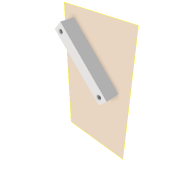
# Autodesk Inventor part: NematostellaImager_mirrormount
Saved by Autodesk Inventor 2022.5 (Build 265521000, 521)
## iProperties
Created: 2023-11-06
Part Number: NematostellaImager_mirrormount
Material: Generisch
Document SubType Name: Modeling
Designer: diederichbenedict
Density: 1 g/cm^3
Appearance: Vorgabe
Author: diederichbenedict
Autodesk Inventor part; units mm, degrees
ref_plane "YZ Plane" through (0, 0, 0) normal (1, 0, 0) x (0, 1, 0)
ref_plane "XZ Plane" through (0, 0, 0) normal (0, 1, 0) x (-1, 0, 0)
ref_plane "XY Plane" through (0, 0, 0) normal (0, 0, 1) x (1, 0, 0)
ref_plane "Arbeitsebene1" through (0, 0, 0) normal (0, 0, 1) x (1, 0, 0)
sketch "Skizze1" plane through (0, 0, 0) normal (0, 0, 1) x (1, 0, 0)
  line L0 (-0.2844, 28.5315) -> (-56.8529, 85.1) projected
  circle A0 centre (-11.3693, 45.2732) radius 1.49 projected
  circle A1 centre (-41.3693, 75.2732) radius 1.4 projected
  line L1 (-47.0261, 75.2732) -> (-41.3693, 80.9301)
  line L2 (-41.3693, 80.9301) -> (-5.7124, 45.2732)
  line L3 (-5.7124, 45.2732) -> (-11.3693, 39.6164)
  line L4 (-11.3693, 39.6164) -> (-47.0261, 75.2732)
  point P0 (0, 0)
  dimension "d0" = 4
  dimension "d1" = 4
  dimension "d2" = 4
  dimension "d3" = 4
  constraints: 8 end point, 2 parallel, 2 perpendicular, 1 point on line
  measures "d0" distance from line of A0.centre L0
  measures "d1" distance from line of A0.centre L2
  measures "d2" distance from line of A0.centre L3
  measures "d3" distance from line of A1.centre L1
extrude "Extrusion1" add sketch "Skizze1" along normal blind 10
